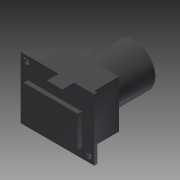
# Autodesk Inventor part: camera_prz
Saved by Autodesk Inventor 2015 SP1 (Build 190203100, 203)
## iProperties
Created: 2015-08-07
Part Number: camera_prz
Material: Generic
Document SubType Name: Modeling
Designer: Alexandre Cherpillod
Mass: 21 g
Surface Area: 29.479 cm^2
Volume: 7.32303 cm^3
Density: 2.86767 g/cm^3
Appearance: Smooth - Black
Author: Alexandre Cherpillod
Autodesk Inventor part; units mm, degrees
ref_plane "YZ Plane" through (0, 0, 0) normal (1, 0, 0) x (0, 1, 0)
ref_plane "XZ Plane" through (0, 0, 0) normal (0, 1, 0) x (-1, 0, 0)
ref_plane "XY Plane" through (0, 0, 0) normal (0, 0, 1) x (1, 0, 0)
sketch "Sketch1" plane through (0, 0, 0) normal (0, 1, 0) x (-1, 0, 0)
  line L0 (0, 0) -> (26.25, 0)
  line L1 (26.25, 0) -> (26.25, -22)
  line L2 (26.25, -22) -> (0, -22)
  line L3 (0, -22) -> (0, 0)
  circle A0 centre (2, -20) radius 0.95
  circle A1 centre (24.25, -2) radius 1
  dimension "d0" = 26.25
  dimension "d1" = 22
  dimension "d3" = 1.9
  dimension "d6" = 2
  dimension "d18" = 2
  dimension "d19" = 2
  dimension "d20" = 2
  dimension "d21" = 2
  constraints: 8 end point, 2 centre point, 2 parallel, 1 horizontal, 1 perpendicular
  measures "d0" distance of L1.end L2.end
  measures "d1" distance of L0.end L1.end
  measures "d3" diameter of A0
  measures "d6" diameter of A1
  measures "d18" distance from line of L1 A1.centre
  measures "d19" distance from line of L0 A1.centre
  measures "d20" distance from line of L3 A0.centre
  measures "d21" distance from line of L2 A0.centre
extrude "Extrusion1" add sketch "Sketch1" along normal blind 1.1
sketch "Sketch2" plane through (0, 1.1, 0) normal (0, 1, 0) x (1, 0, 0)
  line L0 (0, 22) -> (-26.25, 22) projected
  line L1 (0, 0) -> (0, 22) projected
  line L2 (-22.625, 2.5) -> (-3.625, 2.5)
  line L3 (-3.625, 2.5) -> (-3.625, 19.5)
  line L4 (-3.625, 19.5) -> (-22.625, 19.5)
  line L5 (-22.625, 19.5) -> (-22.625, 2.5)
  line L6 (-22.625, 2.5) -> (-3.625, 19.5) construction
  line L7 (-3.625, 2.5) -> (-22.625, 19.5) construction
  point P0 (-13.125, 22)
  point P1 (0, 11)
  point P2 (-13.125, 11)
  point P3 (0, 11)
  point P4 (-13.125, 11)
  point P5 (-13.125, 22)
  point P6 (-13.125, 11)
  dimension "d11" = 19
  dimension "d12" = 17
  constraints: 12 end point, 8 midpoint, 2 parallel, 1 horizontal, 1 horizontal alignment, 1 perpendicular, 1 vertical alignment
  measures "d11" distance of L4.end L3.end
  measures "d12" distance of L2.end L3.end
extrude "Extrusion2" add sketch "Sketch2" along normal blind 11.3
sketch "Sketch3" plane through (0, 12.4, 0) normal (0, 1, 0) x (1, 0, 0)
  line L0 (-3.625, 2.5) -> (-3.625, 19.5) construction
  line L1 (-3.625, 19.5) -> (-22.625, 19.5) construction
  line L2 (-22.625, 19.5) -> (-22.625, 2.5) construction
  line L3 (-22.625, 2.5) -> (-3.625, 2.5) construction
  line L4 (-3.625, 19.5) -> (-3.625, 2.5) construction
  circle A0 centre (-13.125, 11) radius 7.5
  point P0 (0, 0)
  point P1 (-13.125, 19.5)
  point P2 (-3.625, 11)
  dimension "d15" = 15
  constraints: 2 midpoint, 1 centre point, 1 coincident
  measures "d15" diameter of A0
extrude "Extrusion3" add sketch "Sketch3" along normal blind 15
sketch "Sketch4" plane through (0, 0, 0) normal (0, -1, 0) x (1, 0, 0)
  line L0 (-7.2, 0) -> (-12.7, 0)
  line L1 (-12.7, 0) -> (-12.7, -3.3)
  line L2 (-12.7, -3.3) -> (-7.2, -3.3)
  line L3 (-7.2, -3.3) -> (-7.2, 0)
  line L4 (0, 0) -> (-26.25, 0) projected
  circle A0 centre (-2, -20) radius 0.95 projected
  dimension "d22" = 5.5
  dimension "d23" = 3.3
  dimension "d28" = 5.2
  constraints: 8 end point, 2 parallel, 1 collinear, 1 horizontal, 1 perpendicular
  measures "d22" distance of L2.end L1.end
  measures "d23" distance of L0.end L1.end
  measures "d28" distance from line of L3 A0.centre
extrude "Extrusion4" add sketch "Sketch4" along normal blind 4.2 contours L3 L2 L1 L0
sketch "Sketch5" plane through (0, 0, 0) normal (0, -1, 0) x (1, 0, 0)
  line L0 (-4.3784, -18.3892) -> (-23.7162, -18.3892)
  line L1 (-23.7162, -18.3892) -> (-23.7162, -7.4432)
  line L2 (-23.7162, -7.4432) -> (-4.3784, -7.4432)
  line L3 (-4.3784, -7.4432) -> (-4.3784, -18.3892)
  point P0 (0, 0)
  constraints: 8 end point, 2 parallel, 1 horizontal, 1 perpendicular
extrude "Extrusion5" add sketch "Sketch5" along normal blind 1.5
body "Solid1"
